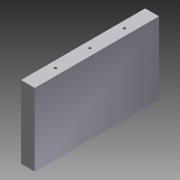
# Autodesk Inventor part: licht_side_simple
Saved by Autodesk Inventor 2015 (Build 190159000, 159)
## iProperties
Created: 2018-01-11
Part Number: licht_side_simple
Material: Generisch
Document SubType Name: Blech
Designer: schueler
Density: 1 g/cm^3
Sheet Metal Rule: Standard_mm
Appearance: Vorgabe
Author: schueler
Autodesk Inventor part; units mm, degrees
ref_plane "YZ Plane" through (0, 0, 0) normal (1, 0, 0) x (0, 1, 0)
ref_plane "XZ Plane" through (0, 0, 0) normal (0, 1, 0) x (-1, 0, 0)
ref_plane "XY Plane" through (0, 0, 0) normal (0, 0, 1) x (1, 0, 0)
sketch "Skizze1" plane through (0, 0, 0) normal (1, 0, 0) x (0, 1, 0)
  line L0 (0, 0) -> (144, 0)
  line L1 (144, 0) -> (144, -84)
  line L2 (144, -84) -> (0, -84)
  line L3 (0, -84) -> (0, 0)
  dimension "d0" = 144
  dimension "d1" = 84
  constraints: 8 end point, 2 parallel, 1 horizontal, 1 perpendicular
  measures "d0" distance of L1.end L2.end
  measures "d1" distance of L0.end L1.end
extrude "Extrusion1" add sketch "Skizze1" along normal blind 16
sketch "Skizze2" plane through (0, 0, 0) normal (0, 0, 1) x (1, 0, 0)
  line L0 (0, 0) -> (0, 144) construction
  line L1 (0, 72) -> (16, 72) construction
  line L2 (16, 144) -> (16, 0) construction
  line L3 (0, 144) -> (16, 144) construction
  line L4 (8, 144) -> (8, 0) construction
  line L5 (0, 144) -> (16, 144) construction
  line L6 (0, 0) -> (16, 0) construction
  line L7 (0, 144) -> (16, 144) construction
  line L8 (16, 144) -> (16, 0) construction
  line L9 (16, 0) -> (0, 0) construction
  line L10 (0, 0) -> (0, 144) construction
  line L11 (0, 112) -> (16, 112) construction
  line L12 (0, 32) -> (16, 32) construction
  point P0 (8, 112)
  point P1 (8, 72)
  point P2 (8, 32)
  dimension "d4" = 40
  dimension "d5" = 40
  constraints: 16 end point, 6 midpoint, 4 point on line, 3 perpendicular, 2 parallel, 1 horizontal, 1 vertical
  measures "d4" distance of L1.end L11.end
  measures "d5" distance of L1.end L12.end
hole "Bohrung1" at (8, 112, 0) at (8, 72, 0) at (8, 32, 0) direction (0, 0, -1) diameter 3 depth 30 tip angle 118
sketch "Skizze3" plane through (0, 144, 0) normal (0, 1, 0) x (1, 0, 0)
  line L0 (0, 0) -> (16, 0)
  line L1 (16, 0) -> (16, 84)
  line L2 (16, 84) -> (0, 84)
  line L3 (0, 84) -> (0, 0)
  line L4 (8, 0) -> (8, 84) construction
  line L5 (0, 84) -> (16, 84) construction
  line L6 (16, 0) -> (16, 84) construction
  line L7 (16, 42) -> (0, 42) construction
  line L8 (0, 84) -> (0, 0) construction
  line L9 (0, 14) -> (16, 14) construction
  line L10 (0, 64) -> (16, 64) construction
  point P0 (8, 14)
  point P1 (8, 64)
  dimension "d13" = 20
  dimension "d14" = 50
  constraints: 16 end point, 6 midpoint, 4 point on line, 3 parallel, 2 perpendicular, 1 horizontal
  measures "d13" distance of L2.end L10.start
  measures "d14" distance of L9.start L10.start
hole "Bohrung2" at (8, 144, -14) at (8, 144, -64) direction (0, -1, 0) diameter 3 depth 25 tip angle 118
equation "\"Biegeradius\" = Stärke"
equation "\"BreiteBiegungsfreistellung\" = Stärke"
equation "\"TiefeBiegungsfreistellung\" = 0.5 * Stärke"
equation "\"GrößeEckenfreistellung\" = 4 * Stärke"
equation "\"MinimalRest\" = 2 * Stärke"
equation "\"Übergangsradius\" = Biegeradius"
equation "\"JacobiRadiusGröße\" = Biegeradius"
equation "\"Abstandsgröße\" = Stärke"
equation "\"Stärke\" = 0.5"
